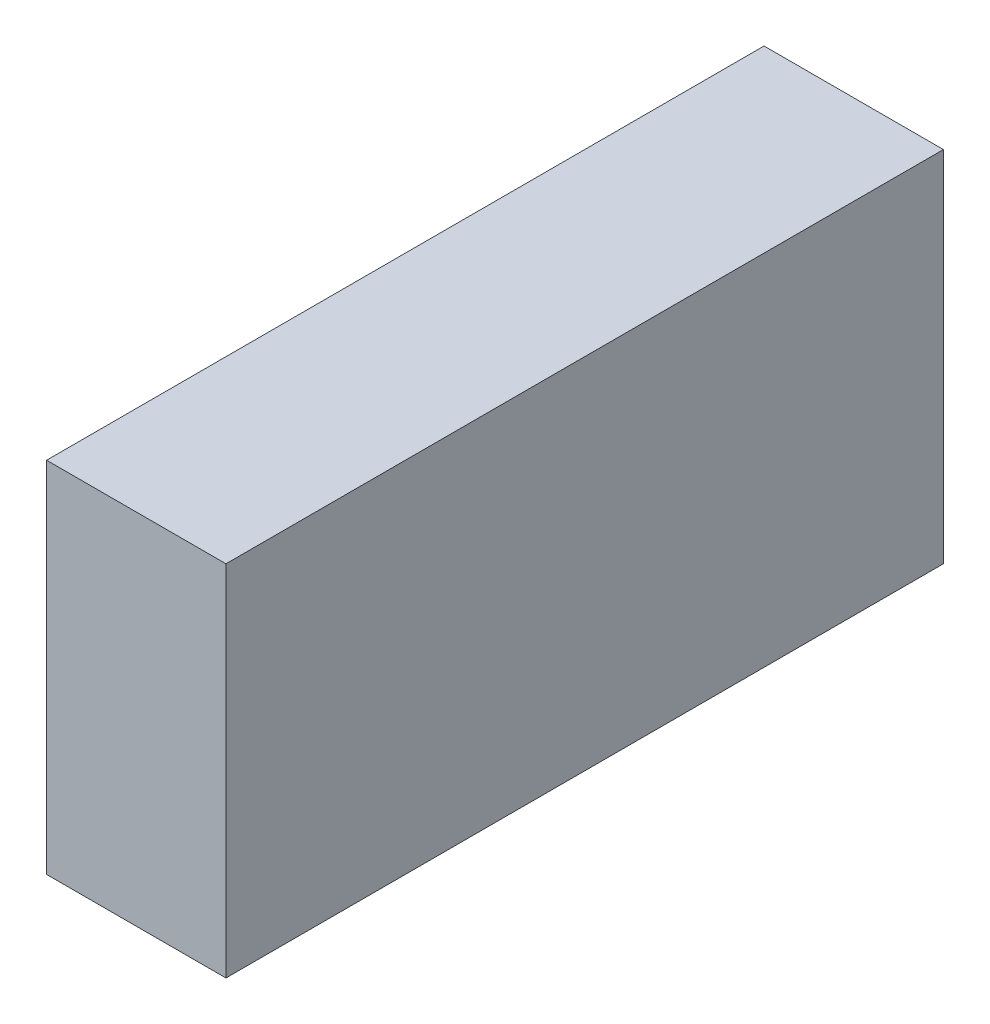
# Autodesk Inventor part: slot1
Saved by Autodesk Inventor 2022 (Build 260153000, 153)
## iProperties
Created: 2022-03-14
Part Number: slot1
Material: Generic
Document SubType Name: Modeling
Designer: br4ch
Density: 1 g/cm^3
Appearance: Default
Author: br4ch
Autodesk Inventor part; units mm, degrees
ref_plane "YZ Plane" through (0, 0, 0) normal (1, 0, 0) x (0, 1, 0)
ref_plane "XZ Plane" through (0, 0, 0) normal (0, 1, 0) x (-1, 0, 0)
ref_plane "XY Plane" through (0, 0, 0) normal (0, 0, 1) x (1, 0, 0)
sketch "Sketch1" plane through (0, 0, 0) normal (1, 0, 0) x (0, 1, 0)
  line L0 (4, 10) -> (-6, 10)
  line L1 (-6, 10) -> (-6, -10)
  line L2 (-6, -10) -> (4, -10)
  line L3 (4, -10) -> (4, 10)
  point P0 (0, 0)
  dimension "d0" = 10
  constraints: 8 end point, 2 parallel, 1 horizontal, 1 perpendicular
  measures "d0" distance of L2.end L1.end
extrude "Extrusion1" add sketch "Sketch1" along normal blind 5
body "Solid1"
